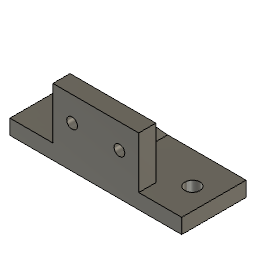
HalterungLinearfuehrung (Autodesk Fusion 360 design; units mm, degrees)
part number: 2025-11-18-11-24-42-761
Autodesk Fusion 360 part; units mm, degrees
sketch "Skizze1" plane through (0, 0, 0) normal (0, 0, 1) x (1, 0, 0)
  line L0 (0, 0) -> (80, 0)
  line L1 (80, 0) -> (80, 30)
  line L2 (80, 30) -> (0, 30)
  line L3 (0, 30) -> (0, 0)
  line L4 (0, 30) -> (10, 30)
  line L5 (10, 30) -> (10, 15)
  line L6 (10, 15) -> (0, 15)
  line L7 (0, 15) -> (0, 30)
  line L8 (80, 30) -> (70, 30)
  line L9 (70, 30) -> (70, 15)
  line L10 (70, 15) -> (80, 15)
  line L11 (80, 15) -> (80, 30)
  circle A0 centre (10, 15) radius 3.5
  circle A1 centre (70, 15) radius 3.5
  dimension "d1" = 80
  dimension "d2" = 30
  dimension "d3" = 10
  dimension "d4" = 15
  dimension "d5" = 10
  dimension "d6" = 15
  dimension "d7" = 7
  dimension "d8" = 7
  constraint horizontal L0
  constraint vertical L1
  constraint horizontal L2
  constraint vertical L3
  constraint coincident L0.start L3.end
  constraint horizontal L4
  constraint vertical L5
  constraint horizontal L6
  constraint vertical L7
  constraint horizontal L8
  constraint vertical L9
  constraint horizontal L10
  constraint vertical L11
  constraint coincident L5.end L6.start
  constraint coincident L9.end L10.start
  measures "d1" distance of L0.start L0.end
  measures "d2" distance of L0.start L2.end
  measures "d3" distance of L2.end L4.end
  measures "d4" distance of L2.end L6.end
  measures "d5" distance of L1.end L8.end
  measures "d6" distance of L1.end L10.end
  measures "d7" diameter of A0
  measures "d8" diameter of A1
extrude "Extrusion1" add sketch "Skizze1" along normal blind 7 contours L0 L1 L2 L3 L5 L6 L9 L10 A0 A1 | L2 L3 L4 L5 L6 L7 A0 | L1 L2 L8 L9 L10 L11 A1
sketch "Skizze2" plane through (0, 0, 0) normal (0, 1, 0) x (1, 0, 0)
sketch "Skizze3" plane through (0, 0, 7) normal (0, 0, 1) x (-1, 0, 0)
  circle A0 centre (-70, -15) radius 3.5
  circle A1 centre (-10, -15) radius 3.5
  line L0 (0, -30) -> (0, 0)
  line L1 (0, 0) -> (-80, 0)
  line L2 (-80, 0) -> (-80, -30)
  line L3 (-80, -30) -> (0, -30)
  line L4 (0, 0) -> (-80, 0)
  line L5 (-80, 0) -> (-80, -5)
  line L6 (-80, -5) -> (0, -5)
  line L7 (0, -5) -> (0, 0)
  dimension "d11" = 5
  constraint horizontal L4
  constraint vertical L5
  constraint horizontal L6
  constraint vertical L7
  constraint coincident L0.end L1.start
  measures "d11" distance of L0.end L6.end
extrude "Extrusion2" add sketch "Skizze3" along normal blind 24 contours L0 L1 L2 L4 L5 L6 L7
sketch "Skizze4" plane through (0, 0, 0) normal (0, -1, 0) x (1, 0, 0)
  line L0 (0, 0) -> (80, 0)
  line L1 (80, 0) -> (80, 31)
  line L2 (80, 31) -> (0, 31)
  line L3 (0, 31) -> (0, 0)
  line L4 (40, 31) -> (40, 19)
  line L5 (40, 0) -> (40, 19.5)
  line L6 (40, 19.5) -> (51, 19.5)
  circle A0 centre (51, 19.5) radius 2.5
  line L7 (40, 19.5) -> (29, 19.5)
  circle A1 centre (29, 19.5) radius 2.5
  dimension "d37" = 19.5
  dimension "d38" = 11
  dimension "d39" = 5
  dimension "d40" = 11
  dimension "d41" = 5
  constraint midpoint L2 L4.start
  constraint perpendicular L2 L4
  constraint midpoint L0 L5.start
  constraint perpendicular L4 L6
  constraint coincident L6.end A0.centre
  constraint perpendicular L4 L7
  constraint coincident L7.end A1.centre
  measures "d37" distance of L5.start L5.end
  measures "d38" distance of L5.end L6.end
  measures "d39" diameter of A0
  measures "d40" distance of L5.end L7.end
  measures "d41" diameter of A1
extrude "Extrusion10" cut sketch "Skizze4" against normal blind 9 contours A0 | A1
extrude "Extrusion11" add 1 faces at (8.8333, 5, 19.1667) along direction (0, 1, 0) blind 3
sketch "Skizze8" plane through (80, 0, 0) normal (1, 0, 0) x (0, 1, 0)
  line L0 (0, 0) -> (30, 0)
  line L1 (30, 0) -> (30, 7)
  line L2 (30, 7) -> (8, 7)
  line L3 (8, 7) -> (8, 31)
  line L4 (8, 31) -> (0, 31)
  line L5 (0, 31) -> (0, 0)
  line L6 (0, 31) -> (8, 31)
  line L7 (8, 31) -> (8, 7)
  line L8 (8, 7) -> (0, 7)
  line L9 (0, 7) -> (0, 31)
  constraint horizontal L6
  constraint vertical L7
  constraint horizontal L8
  constraint vertical L9
  constraint coincident L2.end L3.start
  constraint coincident L4.end L5.start
extrude "Extrusion12" cut sketch "Skizze8" against normal blind 20 contours L3 L4 L5 L6 L7 L8 L9
sketch "Skizze9" plane through (0, 0, 0) normal (-1, 0, 0) x (0, -1, 0)
  line L0 (-30, 0) -> (0, 0)
  line L1 (0, 0) -> (0, 31)
  line L2 (0, 31) -> (-8, 31)
  line L3 (-8, 31) -> (-8, 7)
  line L4 (-8, 7) -> (-30, 7)
  line L5 (-30, 7) -> (-30, 0)
  line L6 (0, 31) -> (-8, 31)
  line L7 (-8, 31) -> (-8, 7)
  line L8 (-8, 7) -> (0, 7)
  line L9 (0, 7) -> (0, 31)
  constraint horizontal L6
  constraint vertical L7
  constraint horizontal L8
  constraint vertical L9
  constraint coincident L3.end L4.start
  constraint coincident L1.end L2.start
extrude "Extrusion13" cut sketch "Skizze9" against normal blind 20 contours L1 L2 L3 L6 L7 L8 L9
sketch "Skizze10" plane through (0, 0, 7) normal (0, 0, 1) x (-1, 0, 0)
  circle A0 centre (-10, -15) radius 3.5
  circle A1 centre (-70, -15) radius 3.5
  line L0 (-20, -8) -> (-60, -8)
  line L1 (-60, -8) -> (-60, 0)
  line L2 (-60, 0) -> (-80, 0)
  line L3 (-80, 0) -> (-80, -30)
  line L4 (-80, -30) -> (0, -30)
  line L5 (0, -30) -> (0, 0)
  line L6 (0, 0) -> (-20, 0)
  line L7 (-20, 0) -> (-20, -8)
  line L8 (-40, -30) -> (-36.5, -30)
  line L9 (-36.5, -30) -> (-43.5, -30)
  line L10 (-43.5, -30) -> (-43.5, -8)
  line L11 (-43.5, -8) -> (-36.5, -8)
  line L12 (-36.5, -8) -> (-36.5, -30)
  dimension "d52" = 3.5
  dimension "d53" = 7
  constraint midpoint L4 L8.start
  constraint parallel L4 L8
  constraint horizontal L9
  constraint vertical L10
  constraint horizontal L11
  constraint vertical L12
  measures "d52" distance of L8.start L8.end
  measures "d53" distance of L8.end L9.end
extrude "Extrusion14" add sketch "Skizze10" along normal blind 24 contours L0 L4 L8 L9 L10 L11 L12
chamfer "Fase3" distance 22 distance2 24 1 edges at (40, 30, 31) measured on face at (41.1667, 2.6667, 31)
